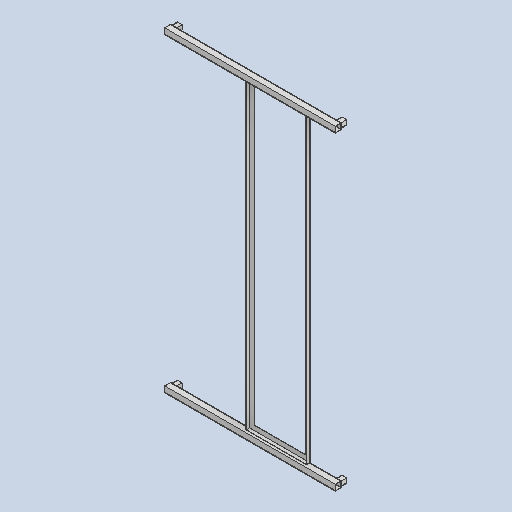
# Autodesk Inventor part: apoioControladora
Saved by Autodesk Inventor 2025 (Build 290162000, 162)
## iProperties
Created: 2022-08-17
Part Number: apoioControladora
Material: Generic
Document SubType Name: Modeling
Designer: cvss2
Density: 1 g/cm^3
Appearance: Default
Author: cvss2
Autodesk Inventor part; units mm, degrees
ref_plane "YZ Plane" through (0, 0, 0) normal (1, 0, 0) x (0, 1, 0)
ref_plane "XZ Plane" through (0, 0, 0) normal (0, 1, 0) x (-1, 0, 0)
ref_plane "XY Plane" through (0, 0, 0) normal (0, 0, 1) x (1, 0, 0)
sketch "Sketch1" plane through (0, 0, 0) normal (0, 0, 1) x (1, 0, 0)
  line L0 (0, 0) -> (-1405, 0)
  line L1 (-1405, 0) -> (-1405, -2605)
  line L2 (-1405, -2605) -> (0, -2605)
  line L3 (0, -2605) -> (0, 0)
  line L4 (-1355, -2555) -> (-1355, -50)
  line L5 (-1355, -50) -> (-50, -50)
  line L6 (-50, -50) -> (-50, -2555)
  line L7 (-50, -2555) -> (-1355, -2555)
  line L8 (-755, -50) -> (-255, -50)
  line L9 (-255, -50) -> (-255, -2555)
  line L10 (-255, -2555) -> (-755, -2555)
  line L11 (-755, -2555) -> (-755, -50)
  line L12 (-295, -2515) -> (-295, -90)
  line L13 (-295, -90) -> (-715, -90)
  line L14 (-715, -90) -> (-715, -2515)
  line L15 (-715, -2515) -> (-295, -2515)
  line L16 (-1355, -2555) -> (-1405, -2555)
  line L17 (-50, -2555) -> (0, -2555)
  line L18 (-50, -50) -> (0, -50)
  line L19 (-1355, -50) -> (-1405, -50)
  point P0 (-755, -2555)
  point P1 (-255, -2555)
  point P2 (-255, -50)
  dimension "d0" = 1405
  dimension "d1" = 2605
  dimension "d2" = 50
  dimension "d3" = 500
  dimension "d4" = 2505
  dimension "d5" = 600
  dimension "d6" = 40
  dimension "d27" = 50
  constraints: 40 end point, 8 parallel, 7 point on line, 6 perpendicular, 2 horizontal, 6 other
  measures "d0" distance of L2.end L1.end
  measures "d1" distance of L1.end L0.end
  measures "d2" distance between parallel lines of L1 L4
  measures "d3" distance of L9.end L10.end
  measures "d4" distance of L8.end L9.end
  measures "d5" distance between parallel lines of L4 L11
  measures "d6" distance between parallel lines of L9 L12
  measures "d27" distance between parallel lines of L2 L7
extrude "Extrusion1" add sketch "Sketch1" along normal blind 50 contours L3 L18 L5 L19 L1 L0 | L3 L2 L1 L16 L7 L17
extrude "Extrusion2" add sketch "Sketch1" along normal blind 30 separate body contours L9 L7 L11 L5
shell "Shell1" thickness 3 removed faces 5 at (-268.3333, -898.3333, 30) at (-575, -90, 10) at (-295, -898.3333, 10) at (-435, -2515, 10) at (-715, -1706.6667, 10) bodies 2
shell "Shell2" thickness 3 removed faces 4 at (-1405, -16.6667, 16.6667) at (-1405, -2571.6667, 16.6667) at (0, -2588.3333, 16.6667) at (0, -33.3333, 16.6667) bodies 1
sketch "Sketch2" plane through (0, 0, 0) normal (0, 0, -1) x (-1, 0, 0)
  line L0 (1405, 0) -> (1405, -50) projected
  line L1 (0, 0) -> (1405, 0) projected
  line L2 (0, -50) -> (0, 0) projected
  line L3 (1405, -50) -> (0, -50) projected
  line L4 (0, -2605) -> (0, -2555) projected
  line L5 (1405, -2605) -> (0, -2605) projected
  line L6 (1405, -2555) -> (1405, -2605) projected
  line L7 (0, -2555) -> (1405, -2555) projected
  line L8 (1405, -50) -> (0, -50) projected
  line L9 (1405, -50) -> (1355, -50)
  line L10 (1355, -50) -> (1355, 0)
  line L11 (1355, 0) -> (1405, 0)
  line L12 (1405, 0) -> (1405, -50)
  line L13 (1360, -5) -> (1360, -45)
  line L14 (1360, -45) -> (1400, -45)
  line L15 (1400, -45) -> (1400, -5)
  line L16 (1400, -5) -> (1360, -5)
  line L17 (1355, -2606) -> (1355, -2556)
  line L18 (1360, -2561) -> (1360, -2601)
  line L19 (1360, -2601) -> (1400, -2601)
  line L20 (1400, -2601) -> (1400, -2561)
  line L21 (1400, -2561) -> (1360, -2561)
  line L22 (1405, -2606) -> (1355, -2606)
  line L23 (1355, -2556) -> (1405, -2556)
  line L24 (1405, -2556) -> (1405, -2606)
  line L25 (-1, -50) -> (-1, 0)
  line L26 (4, -5) -> (4, -45)
  line L27 (4, -45) -> (44, -45)
  line L28 (44, -45) -> (44, -5)
  line L29 (44, -5) -> (4, -5)
  line L30 (49, -50) -> (-1, -50)
  line L31 (-1, 0) -> (49, 0)
  line L32 (49, 0) -> (49, -50)
  line L33 (-1, -2606) -> (-1, -2556)
  line L34 (4, -2561) -> (4, -2601)
  line L35 (4, -2601) -> (44, -2601)
  line L36 (44, -2601) -> (44, -2561)
  line L37 (44, -2561) -> (4, -2561)
  line L38 (49, -2606) -> (-1, -2606)
  line L39 (-1, -2556) -> (49, -2556)
  line L40 (49, -2556) -> (49, -2606)
  point P0 (49, 0)
  dimension "d13" = 50
  dimension "d14" = 50
  dimension "d15" = 5
  dimension "d18" = 2556
  dimension "d21" = 1356
  constraints: 64 end point, 4 parallel, 2 horizontal, 2 perpendicular, 1 vertical, 54 other
  measures "d13" distance of L10.end L11.end
  measures "d14" distance of L9.end L10.end
  measures "d15" distance between parallel lines of L10 L13
  measures "d18" distance of L10.end L17.end
  measures "d21" distance of L10.end L25.end
extrude "Extrusion3" add sketch "Sketch2" along normal blind 50 separate body contours L16 L15 L14 L13 | L21 L20 L19 L18 | L29 L28 L27 L26 | L37 L36 L35 L34
shell "Shell3" thickness 3 removed faces 4 at (-1386.6667, -31.6667, -50) at (-1373.3333, -2574.3333, -50) at (-17.3333, -2574.3333, -50) at (-30.6667, -18.3333, -50) bodies 3
equation "\"d4\" = d1 - 2 * d27"
body "Solid1"
body "Solid2"
body "Solid3"
